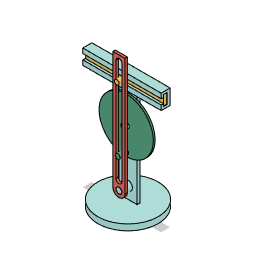
Crank and Slotted Link Mechanism (Autodesk Fusion 360 design; units mm, degrees)
Autodesk Fusion 360 part; units mm, degrees
note: some values were not read from the file. Set by a fixed rule: which face or edge a step refers to.
sketch "Holder stand" plane through (0, 0, 0) normal (0, 1, 0) x (1, 0, 0)
  circle A0 centre (0, 0) radius 50
  dimension "d1" = 100
  constraint coincident A0.centre origin
  measures "d1" diameter of A0
extrude "Extrude1" add sketch "Holder stand" along normal blind 10 makes body 1
sketch "Holder" plane through (0, 10, 0) normal (0, 1, 0) x (-1, 0, 0)
  circle A0 centre (0, 0) radius 50
  line L0 (0, 0) -> (-15, 0)
  line L1 (-15, 0) -> (-15, -5)
  line L2 (-15, -5) -> (0, -5)
  line L3 (0, 0) -> (15, 0)
  line L4 (15, -5) -> (0, -5)
  line L5 (15, 0) -> (15, -5)
  constraint horizontal L0
  constraint vertical L1
  constraint horizontal L2
  constraint coincident A0.centre L0.start
extrude "Extrude2" cut sketch "Holder" against normal blind 40 contours L0 L1 L2 L3 L4 L5 bodies 1
extrude "Extrude3" add sketch "Holder" along normal blind 190 separate body contours L0 L1 L2 L3 L4 L5 makes body 2
extrude "Extrude4" add sketch "Holder" against normal up to surface (10 mm away) contours L0 L1 L2 L3 L4 L5 bodies 2
sketch "Crank holder" plane through (0, 0, 0) normal (0, 0, 1) x (1, 0, 0)
  line L0 (15, 0) -> (15, 200)
  line L1 (15, 200) -> (-15, 200)
  line L2 (-15, 200) -> (-15, 0)
  line L3 (-15, 0) -> (15, 0)
  line L4 (0, 200) -> (0, 118)
  circle A0 centre (0, 118) radius 5
  dimension "d11" = 82
  dimension "d12" = 10
  constraint midpoint L1 L4.start
  constraint perpendicular L1 L4
  constraint coincident L4.end A0.centre
  measures "d11" distance of L4.start L4.end
  measures "d12" diameter of A0
extrude "Extrude5" add sketch "Crank holder" along normal blind 7 contours A0 bodies 2
sketch "Crank" plane through (0, 0, 0) normal (0, 0, 1) x (1, 0, 0)
  circle A0 centre (0, 118) radius 5
  line L0 (15, 0) -> (15, 200)
  line L1 (15, 200) -> (-15, 200)
  line L2 (-15, 200) -> (-15, 0)
  line L3 (-15, 0) -> (15, 0)
  circle A1 centre (0, 118) radius 45
  dimension "d15" = 90
  constraint concentric A0 A1
  measures "d15" diameter of A1
extrude "Extrude6" add sketch "Crank" along normal blind 3 separate body contours A0 | L0 L2 A1 | L0 A1 | L2 A1 makes body 3
extrude "Extrude7" cut sketch "Crank holder" along normal blind 7 contours A0 bodies 3
move_face "OffsetFaces1" offset -0.3 1 faces at (4.9752, 118.4978, 4.6667) on bodies 2
sketch "Slider holder right" plane through (15, 0, 0) normal (1, 0, 0) x (0, 0, -1)
  line L0 (5, 0) -> (5, 200)
  line L1 (5, 200) -> (0, 200)
  line L2 (0, 200) -> (0, 0)
  line L3 (0, 0) -> (5, 0)
  line L4 (0, 200) -> (5, 200)
  line L5 (5, 200) -> (5, 175)
  line L6 (5, 175) -> (0, 175)
  line L7 (0, 175) -> (0, 200)
  dimension "d21" = 25
  constraint horizontal L4
  constraint vertical L5
  constraint horizontal L6
  constraint vertical L7
  constraint coincident L1.end L2.start
  measures "d21" distance of L1.end L6.end
sketch "Slider holder left" plane through (-15, 0, 0) normal (-1, 0, 0) x (0, 0, 1)
  line L0 (0, 0) -> (0, 200)
  line L1 (0, 200) -> (-5, 200)
  line L2 (-5, 200) -> (-5, 0)
  line L3 (-5, 0) -> (0, 0)
  line L4 (-5, 200) -> (0, 200)
  line L5 (0, 200) -> (0, 175)
  line L6 (0, 175) -> (-5, 175)
  line L7 (-5, 175) -> (-5, 200)
  constraint horizontal L4
  constraint vertical L5
  constraint horizontal L6
  constraint vertical L7
  constraint coincident L0 L5.end
  constraint coincident L1.end L2.start
extrude "Extrude8" add sketch "Slider holder right" along normal blind 50 contours L0 L1 L2 L4 L5 L6 L7 bodies 2
extrude "Extrude9" add sketch "Slider holder left" along normal blind 50 contours L0 L1 L2 L4 L5 L6 L7 bodies 2
sketch "Slider holder front" plane through (0, 0, 0) normal (0, 0, 1) x (1, 0, 0)
  circle A0 centre (0, 118) radius 4.7
  line L0 (15, 0) -> (15, 175)
  line L1 (15, 175) -> (65, 175)
  line L2 (65, 175) -> (65, 200)
  line L3 (65, 200) -> (-65, 200)
  line L4 (-65, 200) -> (-65, 175)
  line L5 (-65, 175) -> (-15, 175)
  line L6 (-15, 175) -> (-15, 0)
  line L7 (-15, 0) -> (15, 0)
  line L8 (-65, 200) -> (65, 200)
  line L9 (65, 200) -> (65, 196)
  line L10 (65, 196) -> (-65, 196)
  line L11 (-65, 196) -> (-65, 200)
  line L12 (-65, 175) -> (65, 175)
  line L13 (65, 175) -> (65, 179)
  line L14 (65, 179) -> (-65, 179)
  line L15 (-65, 179) -> (-65, 175)
  dimension "d26" = 4
  dimension "d27" = 4
  constraint horizontal L8
  constraint vertical L9
  constraint horizontal L10
  constraint vertical L11
  constraint coincident L3.end L4.start
  constraint horizontal L12
  constraint vertical L13
  constraint horizontal L14
  constraint vertical L15
  constraint coincident L2 L13.end
  constraint coincident L4.end L5.start
  measures "d26" distance of L3.end L10.end
  measures "d27" distance of L4.end L14.end
extrude "Extrude10" add sketch "Slider holder front" along normal blind 10 contours L1 L2 L4 L5 L12 L13 L14 L15 | L2 L3 L4 L8 L9 L10 L11 bodies 2
sketch "Slider barrier bottom" plane through (0, 179, 0) normal (0, 1, 0) x (-1, 0, 0)
  line L0 (-65, 0) -> (65, 0)
  line L1 (65, 0) -> (65, 10)
  line L2 (65, 10) -> (-65, 10)
  line L3 (-65, 10) -> (-65, 0)
  line L4 (65, 10) -> (-65, 10)
  line L5 (-65, 10) -> (-65, 6)
  line L6 (-65, 6) -> (65, 6)
  line L7 (65, 6) -> (65, 10)
  dimension "d30" = 4
  constraint horizontal L4
  constraint vertical L5
  constraint horizontal L6
  constraint vertical L7
  constraint coincident L1.end L2.start
  measures "d30" distance of L1.end L6.end
sketch "Slider barrier top" plane through (0, 196, 0) normal (0, -1, 0) x (1, 0, 0)
  line L0 (-65, 0) -> (65, 0)
  line L1 (65, 0) -> (65, 10)
  line L2 (65, 10) -> (-65, 10)
  line L3 (-65, 10) -> (-65, 0)
  line L4 (-65, 10) -> (65, 10)
  line L5 (65, 10) -> (65, 6)
  line L6 (65, 6) -> (-65, 6)
  line L7 (-65, 6) -> (-65, 10)
  dimension "d31" = 4
  constraint horizontal L4
  constraint vertical L5
  constraint horizontal L6
  constraint vertical L7
  constraint coincident L2.end L3.start
  measures "d31" distance of L2.end L6.end
extrude "Extrude11" add sketch "Slider barrier top" along normal blind 4 contours L1 L2 L3 L4 L5 L6 L7 bodies 2
extrude "Extrude12" add sketch "Slider barrier bottom" along normal blind 4 contours L1 L2 L3 L4 L5 L6 L7 bodies 2
sketch "Slider" plane through (65, 0, 0) normal (1, 0, 0) x (0, 0, -1)
  line L0 (-10, 175) -> (5, 175)
  line L1 (5, 175) -> (5, 200)
  line L2 (5, 200) -> (-10, 200)
  line L3 (-10, 200) -> (-10, 192)
  line L4 (-10, 192) -> (-6, 192)
  line L5 (-6, 192) -> (-6, 196)
  line L6 (-6, 196) -> (0, 196)
  line L7 (0, 196) -> (0, 179)
  line L8 (0, 179) -> (-6, 179)
  line L9 (-6, 179) -> (-6, 183)
  line L10 (-6, 183) -> (-10, 183)
  line L11 (-10, 183) -> (-10, 175)
  line L12 (-6, 196) -> (0, 196)
  line L13 (0, 196) -> (0, 179)
  line L14 (0, 179) -> (-6, 179)
  line L15 (-6, 179) -> (-6, 196)
  constraint horizontal L12
  constraint vertical L13
  constraint horizontal L14
  constraint vertical L15
  constraint coincident L7.end L8.start
  constraint coincident L5.end L6.start
extrude "Extrude13" add sketch "Slider" against normal blind 130 separate body contours L5 L6 L7 L8 L9 L12 L13 L14 L15 makes body 4
move_face "OffsetFaces2" offset -0.3 8 faces at (65, 186, 2) (21.6667, 196, 4) (-21.6667, 190.3333, 0) (-65, 186, 2) (21.6667, 186, 6) (-21.6667, 193.3333, 6) (-21.6667, 180.3333, 6) (21.6667, 179, 2) on bodies 4
sketch "Link holder" plane through (0, 0, 0) normal (0, 0, 1) x (1, 0, 0)
  line L0 (15, 175) -> (-15, 175)
  line L1 (-15, 175) -> (-15, 0)
  line L2 (-15, 0) -> (15, 0)
  line L3 (15, 0) -> (15, 175)
  circle A0 centre (0, 118) radius 4.7
  circle A1 centre (0, 30) radius 5
  dimension "d39" = 10
  measures "d39" diameter of A1
extrude "Extrude14" add sketch "Link holder" along normal blind 15 contours A1 bodies 2
sketch "Slotted link" plane through (0, 0, 15) normal (0, 0, 1) x (1, 0, 0)
  circle A0 centre (0, 30) radius 5
  circle A1 centre (0, 30) radius 10
  line L0 (-10, 30) -> (10, 30)
  line L1 (-10, 30) -> (10, 30)
  line L2 (10, 30) -> (10, 225)
  line L3 (10, 225) -> (-10, 225)
  line L4 (-10, 225) -> (-10, 30)
  line L5 (-5, 30) -> (5, 30)
  line L6 (5, 30) -> (5, 220)
  line L7 (5, 220) -> (-5, 220)
  line L8 (-5, 220) -> (-5, 30)
  circle A2 centre (0, 45) radius 5
  circle A3 centre (0, 215) radius 5
  dimension "d42" = 5
  constraint coincident A1 L0.start
  constraint coincident A1 L0.end
  constraint horizontal L0
  constraint horizontal L1
  constraint vertical L2
  constraint horizontal L3
  constraint vertical L4
  constraint horizontal L5
  constraint vertical L6
  constraint horizontal L7
  constraint vertical L8
  constraint coincident L1 L5.start
  constraint coincident A0 L5.start
  constraint tangent L7 A3
  measures "d42" distance of A0
extrude "Extrude15" add sketch "Slotted link" against normal blind 4 separate body contours A0 A1 L0 L1 | A1 L0 L1 L6 | A0 A1 L6 L8 | A1 L0 L1 L8 | A1 L2 L3 L4 L6 L7 L8 | A1 L6 A2 | A1 L8 A2 | L6 L7 A3 | L7 L8 A3 makes body 5
move_face "OffsetFaces3" offset -0.3 1 faces at (4.9752, 29.5022, 10) on bodies 2
sketch "Slotted link holder" plane through (0, 0, 15) normal (0, 0, 1) x (1, 0, 0)
  circle A0 centre (0, 30) radius 4.7
  circle A1 centre (0, 30) radius 7.5
  dimension "d46" = 15
  constraint concentric A0 A1
  measures "d46" diameter of A1
extrude "Extrude16" add sketch "Slotted link holder" along normal blind -15 and the other way blind 4 bodies 2
sketch "Crank pin" plane through (0, 0, 3) normal (0, 0, 1) x (1, 0, 0)
  circle A0 centre (0, 118) radius 5
  circle A1 centre (0, 118) radius 45
  circle A2 centre (0, 80) radius 4
  dimension "d51" = 8
  measures "d51" diameter of A2
sketch "slider pin" plane through (0, 0, 5.7) normal (0, 0, 1) x (1, 0, 0)
  line L0 (64.7, 179.3) -> (64.7, 195.7)
  line L1 (64.7, 195.7) -> (-64.7, 195.7)
  line L2 (-64.7, 195.7) -> (-64.7, 179.3)
  line L3 (-64.7, 179.3) -> (64.7, 179.3)
  circle A0 centre (0, 187.6038) radius 4
  dimension "d52" = 8
  measures "d52" diameter of A0
extrude "Extrude17" add sketch "slider pin" along normal blind 13 contours A0 bodies 4
extrude "Extrude18" add sketch "Crank pin" along normal blind 14 contours A2 bodies 3
copy_body "Body->Comp1" bodies 1 removing the originals makes body 6 in component "Holder stand"
copy_body "Body->Comp2" bodies 2 removing the originals makes body 7 in component "Holder"
copy_body "Body->Comp3" bodies 3 removing the originals makes body 8 in component "Crank"
copy_body "Body->Comp4" bodies 5 removing the originals makes body 9 in component "Slotted link"
copy_body "Body->Comp5" bodies 4 removing the originals makes body 10 in component "Slider"
component "Holder stand" placed x (1, 0, 0) y (0, 1, 0) z (0, 0, 1) at (0, 0, 0)
component "Holder" placed x (1, 0, 0) y (0, 1, 0) z (0, 0, 1) at (0, 0, 0)
component "Crank" placed x (1, 0, 0) y (0, 1, 0) z (0, 0, 1) at (0, 0, 0)
component "Slotted link" placed x (1, 0, 0) y (0, 1, 0) z (0, 0, 1) at (0, 0, 0)
component "Slider" placed x (1, 0, 0) y (0, 1, 0) z (0, 0, 1) at (0, 0, 0)
named bodies: "Holder stand", "Holder", "Crank", "Slider", "Slotted link"
